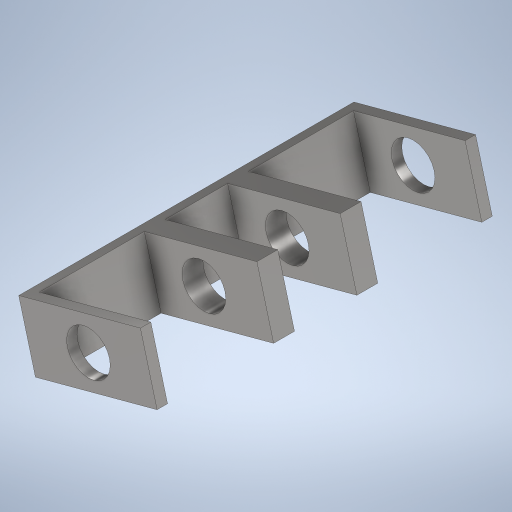
# Autodesk Inventor part: Suwak chwytaka
Saved by Autodesk Inventor 2024.1 (Build 281209000, 209)
## iProperties
Created: 2024-05-28
Part Number: Suwak chwytaka
Material: Stal, węglowa
Document SubType Name: Modeling
Designer: Krzysiu
Density: 7.85 g/cm^3
Appearance: Częściowo polerowany
Stock Number: 05
Mass: 4.17552 g
Surface Area: 11.3145 cm^2
Volume: 0.531913 cm^3
Author: Krzysiu
Autodesk Inventor part; units mm, degrees
ref_plane "YZ Plane" through (0, 0, 0) normal (1, 0, 0) x (0, 1, 0)
ref_plane "XZ Plane" through (0, 0, 0) normal (0, 1, 0) x (-1, 0, 0)
sketch "Szkic1" plane through (0, 0, 0) normal (0, 0, 1) x (1, 0, 0)
  line L0 (0, 0) -> (-25, 0)
  line L1 (-25, 0) -> (-17.2354, -28.9778)
  line L2 (-25, 0) -> (5, 0) construction
  line L3 (-25, 0) -> (-34.8351, 36.7052)
  line L4 (-25, 0) -> (13, 0) construction
  line L5 (-34.8351, 36.7052) -> (-34.8351, 54.7052)
  line L6 (-34.8351, 54.7052) -> (0, 54.7052)
  line L7 (-34.8351, 54.7052) -> (-24.8351, 72.0257)
  line L8 (-34.8351, 54.7052) -> (-14.8351, 54.7052) construction
  line L9 (-34.8351, 54.7052) -> (-24.8351, 37.3847)
  line L10 (-34.8351, 54.7052) -> (-14.8351, 54.7052) construction
  circle A0 centre (-25, 0) radius 1.5
  line L11 (0, 0) -> (0, -12)
  line L12 (0, -12) -> (-25, -12)
  line L13 (-25, -12) -> (-17.2354, -28.9778)
  line L14 (-25, -12) -> (-45.5171, 32.862)
  line L15 (-45.5171, 32.862) -> (-48.5127, 50.611)
  line L16 (-45.5171, 32.862) -> (-27.5171, 32.862) construction
  line L17 (-48.5127, 50.611) -> (-35.7696, 35.1962)
  line L18 (-48.5127, 50.611) -> (-28.5127, 50.611) construction
  line L19 (-48.5127, 50.611) -> (-41.5347, 69.3542)
  line L20 (-48.5127, 50.611) -> (-28.5127, 50.611) construction
  circle A1 centre (-25, -12) radius 1.5
  line L21 (-17.2354, -28.9778) -> (2.5, -28.9778)
  circle A2 centre (-17.2354, -28.9778) radius 2.5
  line L22 (-19.7354, -28.9778) -> (-24.7354, -28.9778)
  line L23 (19.7354, -28.9778) -> (24.7354, -28.9778)
  circle A3 centre (17.2354, -28.9778) radius 2.5
  line L24 (25, -12) -> (17.2354, -28.9778)
  line L25 (17.2354, -28.9778) -> (2.5, -28.9778)
  line L26 (0, -12) -> (25, -12)
  line L27 (34.8351, 54.7052) -> (24.8351, 37.3847)
  line L28 (34.8351, 36.7052) -> (34.8351, 54.7052)
  line L29 (48.5127, 50.611) -> (35.7696, 35.1962)
  line L30 (45.5171, 32.862) -> (48.5127, 50.611)
  line L31 (45.5171, 32.862) -> (27.5171, 32.862) construction
  circle A4 centre (25, 0) radius 1.5
  line L32 (25, 0) -> (34.8351, 36.7052)
  circle A5 centre (25, -12) radius 1.5
  line L33 (25, -12) -> (45.5171, 32.862)
  line L34 (0, 0) -> (25, 0)
  line L35 (25, 0) -> (17.2354, -28.9778)
  line L36 (25, 0) -> (-5, 0) construction
  line L37 (25, 0) -> (-13, 0) construction
  line L38 (48.5127, 50.611) -> (28.5127, 50.611) construction
  line L39 (48.5127, 50.611) -> (28.5127, 50.611) construction
  line L40 (34.8351, 54.7052) -> (14.8351, 54.7052) construction
  line L41 (34.8351, 54.7052) -> (14.8351, 54.7052) construction
  line L42 (34.8351, 54.7052) -> (0, 54.7052)
  line L43 (48.5127, 50.611) -> (41.5347, 69.3542)
  line L44 (34.8351, 54.7052) -> (24.8351, 72.0257)
  line L45 (-17.2354, -31.4778) -> (-17.2354, -36.4778)
  line L46 (-17.2354, -36.4778) -> (2.5, -36.4778)
  line L47 (-17.2354, -36.4778) -> (-19.7354, -36.4778)
  line L48 (-24.7354, -28.9778) -> (-24.7354, -31.4778)
  line L49 (-17.2354, -26.4778) -> (-17.2354, -21.4778)
  line L50 (-17.2354, -21.4778) -> (-19.7354, -21.4778)
  line L51 (-24.7354, -26.4778) -> (-24.7354, -28.9778)
  line L52 (-17.2354, -21.4778) -> (2.5, -21.4778)
  line L53 (17.2354, -21.4778) -> (19.7354, -21.4778)
  line L54 (25, 0) -> (17.2354, -28.9778)
  line L55 (25, -12) -> (17.2354, -28.9778)
  line L56 (24.7354, -26.4778) -> (24.7354, -28.9778)
  line L57 (17.2354, -26.4778) -> (17.2354, -21.4778)
  line L58 (19.7354, -28.9778) -> (24.7354, -28.9778)
  circle A6 centre (17.2354, -28.9778) radius 2.5
  line L59 (24.7354, -28.9778) -> (24.7354, -31.4778)
  line L60 (17.2354, -36.4778) -> (19.7354, -36.4778)
  line L61 (17.2354, -31.4778) -> (17.2354, -36.4778)
  line L62 (17.2354, -28.9778) -> (-2.5, -28.9778)
  line L63 (17.2354, -36.4778) -> (-2.5, -36.4778)
  line L64 (17.2354, -21.4778) -> (-2.5, -21.4778)
  line L65 (-17.2354, -28.9778) -> (-2.5, -28.9778)
  arc A7 (-19.7354, -21.4778) -> (-24.7354, -26.4778) centre (-19.7354, -26.4778) ccw
  arc A8 (-24.7354, -31.4778) -> (-19.7354, -36.4778) centre (-19.7354, -31.4778) ccw
  arc A9 (24.7354, -26.4778) -> (19.7354, -21.4778) centre (19.7354, -26.4778) ccw
  arc A10 (19.7354, -36.4778) -> (24.7354, -31.4778) centre (19.7354, -31.4778) ccw
  line L66 (0, -12) -> (0, -15)
  line L67 (0, -15) -> (-25, -15)
  line L68 (-17.2354, -28.9778) -> (-25, -15)
  circle A11 centre (-25, 0) radius 2.1
  line L69 (-25.5435, 2.0284) -> (-19.6514, 3.6072)
  line L70 (-25.5435, 2.0284) -> (-31.4357, 0.4496)
  line L71 (-31.4357, 0.4496) -> (-31.6945, 1.4156)
  line L72 (-31.4357, 0.4496) -> (-30.4357, 0.4496) construction
  line L73 (-31.6945, 1.4156) -> (-19.9102, 4.5732)
  line L74 (-19.9102, 4.5732) -> (-19.6514, 3.6072)
  line L75 (-19.6514, 3.6072) -> (-18.3055, -1.4156)
  line L76 (-18.3055, -1.4156) -> (-30.0898, -4.5732)
  line L77 (-30.0898, -4.5732) -> (-31.4357, 0.4496)
  point P0 (0, 0)
  point P1 (0, 0)
  point P2 (2.5, 0)
  point P3 (-24.7354, -36.4778)
  point P4 (-24.7354, -21.4778)
  point P5 (24.7354, -21.4778)
  point P6 (24.7354, -36.4778)
  dimension "d31" = 4.2
  dimension "d0" = 25
  dimension "d1" = 30
  dimension "d2" = 75
  dimension "d3" = 38
  dimension "d4" = 105
  dimension "d5" = 18
  dimension "d6" = 20
  dimension "d7" = 60
  dimension "d8" = 20
  dimension "d9" = 60
  dimension "d10" = 3
  dimension "d11" = 12
  dimension "d12" = 25
  dimension "d13" = 49.331
  dimension "d14" = 18
  dimension "d15" = 99.58
  dimension "d16" = 20
  dimension "d17" = 50.42
  dimension "d18" = 20
  dimension "d19" = 69.58
  dimension "d20" = 3
  dimension "d21" = 5
  dimension "d22" = 5
  dimension "d23" = 5
  dimension "d24" = 5
  dimension "d25" = 5
  dimension "d26" = 5
  dimension "d27" = 5
  dimension "d28" = 5
  dimension "d29" = 3
  dimension "d30" = 25
  dimension "d32" = 6.1
  dimension "d33" = 6.1
  dimension "d35" = 1
  dimension "d36" = 105
  dimension "d37" = 5.2
  dimension "d38" = 12.2
  constraints: 156 end point, 37 symmetric about line, 15 point on line, 14 point on circle, 13 horizontal, 12 perpendicular, 11 coincident, 10 centre point, 8 equal length, 8 tangent, 3 vertical, 1 horizontal alignment, 11 other
  measures "d0" distance of L0.start L0.end
  measures "d1" distance of L0.end L1.end
  measures "d2" angle of L1 L2
  measures "d3" distance of L0.end L3.end
  measures "d4" angle of L4 L3
  measures "d5" distance of L3.end L5.end
  measures "d6" distance of L5.end L7.end
  measures "d7" angle of L8 L7
  measures "d8" distance of L5.end L9.end
  measures "d9" angle of L9 L10
  measures "d10" diameter of A0
  measures "d11" distance of L0.start L11.end
  measures "d12" distance of L11.end L12.end
  measures "d13" distance of L12.end L14.end
  measures "d14" distance of L14.end L15.end
  measures "d15" angle of L16 L15
  measures "d16" distance of L15.end L17.end
  measures "d17" angle of L17 L18
  measures "d18" distance of L15.end L19.end
  measures "d19" angle of L20 L19
  measures "d20" diameter of A1
  measures "d21" diameter of A2
  measures "d22" distance of L22.start L22.end
  measures "d23" distance of L45.start L45.end
  measures "d24" distance of L49.start L49.end
  measures "d25" radius of A7
  measures "d26" radius of A8
  measures "d27" radius of A9
  measures "d28" radius of A10
  measures "d29" distance of L11.end L66.end
  measures "d30" distance of L66.end L67.end
  measures "d32" distance of L69.start L69.end
  measures "d33" distance of L69.start L70.end
  measures "d35" distance of L70.end L71.end
  measures "d36" angle of L72 L71
  measures "d37" distance of L69.end L75.end
  measures "d38" distance of L75.end L76.end
extrude "Wyciągnięcie proste1" add sketch "Szkic1" along normal blind 2 contours A11 L69 L75 L0 | L0 L75 L76 L1 A11 | L70 L14 L73 L3 | L3 L73 L74 L69 | A11 L1 L76 L14 L70 | L70 L71 L73 L14 | L14 L76 L77 L70
sketch "Szkic2" plane through (0, 0, 2) normal (0, 0, 1) x (1, 0, 0)
  line L0 (-31.6945, 1.4156) -> (-30.0898, -4.5732) projected
  line L1 (-31.6945, 1.4156) -> (-30.7286, 1.6744)
  line L2 (-19.9102, 4.5732) -> (-31.6945, 1.4156) projected
  line L3 (-30.7286, 1.6744) -> (-29.1239, -4.3143)
  line L4 (-30.0898, -4.5732) -> (-18.3055, -1.4156) projected
  line L5 (-29.1239, -4.3143) -> (-30.0898, -4.5732)
  line L6 (-30.0898, -4.5732) -> (-31.6945, 1.4156)
  point P0 (0, 0)
  dimension "d41" = 1
  constraints: 8 end point, 3 perpendicular, 2 point on line
  measures "d41" distance of L0.start L1.end
extrude "Wyciągnięcie proste2" add sketch "Szkic2" along normal blind 11.1 and the other way blind 21.1
sketch "Szkic3" plane through (0, 0, 2) normal (0, 0, 1) x (1, 0, 0)
  line L0 (-30.7286, 1.6744) -> (-29.1239, -4.3143) projected
  line L1 (-30.7286, 1.6744) -> (-29.1239, -4.3143)
  line L2 (-29.1239, -4.3143) -> (-18.3055, -1.4156) projected
  line L3 (-29.1239, -4.3143) -> (-18.3055, -1.4156)
  line L4 (-18.3055, -1.4156) -> (-19.9102, 4.5732)
  line L5 (-19.9102, 4.5732) -> (-30.7286, 1.6744)
  circle A0 centre (-25, 0) radius 2.1 projected
  circle A1 centre (-25, 0) radius 2.1
  point P0 (0, 0)
  constraints: 8 end point, 2 collinear, 2 perpendicular, 1 centre point, 1 coincident
ref_plane "Płaszczyzna konstrukcyjna1" through (-30.7286, 1.6744, -8) normal (0, 0, 1) x (0.2588, -0.9659, 0)
extrude "Wyciągnięcie proste3" add sketch "Szkic3" along normal blind 2 from surface at -10
sketch "Szkic5" plane through (-30.7286, 1.6744, 13.1) normal (0.9659, 0.2588, 0) x (0, 0, -1)
  line L0 (0, 0) -> (1, 0)
  line L1 (32.2, 0) -> (0, 0) projected
  line L2 (1, 0) -> (1, -6.2)
  line L3 (0, -6.2) -> (11.1, -6.2) projected
  line L4 (1, -6.2) -> (0, -6.2)
  line L5 (0, -6.2) -> (0, 0)
  line L6 (32.2, 0) -> (32.2, -6.2)
  line L7 (32.2, -6.2) -> (31.2, -6.2)
  line L8 (32.2, -6.2) -> (0, -6.2) projected
  line L9 (31.2, -6.2) -> (31.2, 0)
  line L10 (32.2, 0) -> (31.2, 0)
  point P0 (13.1, -9.5705)
  dimension "d51" = 1
  dimension "d52" = 1
  constraints: 16 end point, 4 point on line, 3 perpendicular, 1 collinear, 1 horizontal, 1 vertical
  measures "d51" distance of L0.start L0.end
  measures "d52" distance of L6.end L7.end
extrude "Wyciągnięcie proste4" add sketch "Szkic5" along normal blind 11.1 contours L0 L2 L3 L5 | L1 L6 L7 L9
sketch "Szkic6" plane through (0, 0, 13.1) normal (0, 0, 1) x (1, 0, 0)
  circle A0 centre (-25, 0) radius 2.1 projected
  circle A1 centre (-25, 0) radius 2.1
  point P0 (0, 0)
  constraints: 1 centre point, 1 coincident
extrude "Wyciągnięcie proste5" cut sketch "Szkic6" against normal through all
